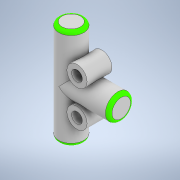
# Autodesk Inventor part: Union Tee 1-8 KQ2T01-00A SMC
Saved by Autodesk Inventor 2021 (Build 250183000, 183)
## iProperties
Created: 2020-07-15
Part Number: Union Tee 1-8 KQ2T01-00A SMC
Material: Generic
Document SubType Name: Modeling
Designer: jgray
Density: 1 g/cm^3
Appearance: Default
Author: jgray
Autodesk Inventor part; units mm, degrees
ref_plane "YZ Plane" through (0, 0, 0) normal (1, 0, 0) x (0, 1, 0)
ref_plane "XZ Plane" through (0, 0, 0) normal (0, 1, 0) x (-1, 0, 0)
ref_plane "XY Plane" through (0, 0, 0) normal (0, 0, 1) x (1, 0, 0)
sketch "Sketch1" plane through (0, 0, 0) normal (0, 1, 0) x (-1, 0, 0)
  circle A0 centre (0, 0) radius 3.75
  dimension "d0" = 7.5
  constraints: 1 centre point, 1 coincident
  measures "d0" diameter of A0
extrude "Extrusion1" add sketch "Sketch1" along normal mid plane 29.8
sketch "Sketch2" plane through (0, 0, 0) normal (1, 0, 0) x (0, 1, 0)
  line L0 (-14.9, 3.75) -> (-14.9, -3.75) projected
  line L1 (14.9, -3.75) -> (14.9, 3.75) projected
  circle A0 centre (0, 0) radius 3.75
  constraints: 1 centre point, 1 coincident
extrude "Extrusion2" add sketch "Sketch2" along normal blind 14.9
sketch "Sketch3" plane through (0, 0, 0) normal (0, 0, 1) x (1, 0, 0)
  line L0 (0, 13.8301) -> (0, -13.8301) construction
  line L1 (-5.2476, 0) -> (14.0163, 0) construction
  circle A0 centre (5.4, 5.4) radius 1.6
  circle A1 centre (5.4, -5.4) radius 1.6
  circle A2 centre (5.4, 5.4) radius 3
  circle A3 centre (5.4, -5.4) radius 3
  point P0 (0, 0)
  point P1 (0, 0)
  dimension "d5" = 5.4
  dimension "d6" = 5.4
  dimension "d7" = 3.2
  dimension "d8" = 3.2
  dimension "d9" = 6
  dimension "d10" = 6
  dimension "d11" = 5.4
  dimension "d12" = 5.4
  constraints: 4 centre point, 4 coincident, 4 end point, 2 midpoint, 2 point on line, 1 horizontal, 1 vertical
  measures "d5" distance from line of point (5.4, 5.4) L1
  measures "d6" distance from line of point (5.4, -5.4) L1
  measures "d7" diameter of A0
  measures "d8" diameter of A1
  measures "d9" diameter of A2
  measures "d10" diameter of A3
  measures "d11" distance from line of A0.centre L0
  measures "d12" distance from line of A1.centre L0
extrude "Extrusion3" add sketch "Sketch3" along normal mid plane 7.4
fillet "Fillet1" radius 1 3 edges at (3.75, 14.9, 0) (14.9, -3.75, 0) (3.75, -14.9, 0)
body "Solid1"
